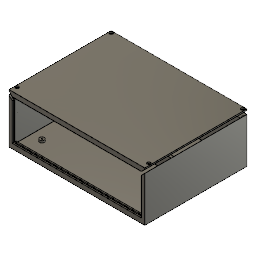
case_v1.26 (Autodesk Fusion 360 design; units mm, degrees)
Autodesk Fusion 360 part; units mm, degrees
sketch "bottom" plane through (0, 0, 0) normal (0, 1, 0) x (1, 0, 0)
  line L0 (-98.8893, -25.3823) -> (99.1107, -25.3823)
  line L1 (99.1107, -25.3823) -> (99.1107, -27.1323)
  line L2 (99.1107, -27.1323) -> (-98.8893, -27.1323)
  line L3 (-98.8893, -27.1323) -> (-98.8893, -25.3823)
  line L4 (-101.3893, 123.8677) -> (101.6107, 123.8677)
  line L5 (101.6107, 123.8677) -> (101.6107, -29.1323)
  line L6 (101.6107, -29.1323) -> (-101.3893, -29.1323)
  line L7 (-101.3893, -29.1323) -> (-101.3893, 123.8677)
  line L8 (-96.3893, 118.8677) -> (96.6107, 118.8677)
  line L9 (96.6107, 118.8677) -> (96.6107, -23.3823)
  line L10 (96.6107, -23.3823) -> (-96.3893, -23.3823)
  line L11 (-96.3893, -23.3823) -> (-96.3893, 118.8677)
  line L12 (96.6107, -23.3823) -> (96.6107, -25.3823)
  line L13 (96.6107, -27.1323) -> (96.6107, -29.1323)
  line L14 (-96.3893, -23.3823) -> (-96.3893, -25.3823)
  line L15 (-96.3893, -27.1323) -> (-96.3893, -29.1323)
  circle A0 centre (-79.3893, -1.6323) radius 3.5
  line L16 (-89.3893, 118.8677) -> (89.6107, 118.8677)
  line L17 (89.6107, 118.8677) -> (89.6107, 56.8677)
  line L18 (89.6107, 56.8677) -> (-89.3893, 56.8677)
  line L19 (-89.3893, 56.8677) -> (-89.3893, 118.8677)
  line L20 (0.1107, 123.8677) -> (0.1107, -29.1323) construction
  line L21 (93.6107, 118.8677) -> (93.6107, 52.8677)
  line L22 (93.6107, 52.8677) -> (-93.3893, 52.8677)
  line L23 (-93.3893, 52.8677) -> (-93.3893, 118.8677)
  circle A1 centre (0.1111, 37.8677) radius 3.5
  line L24 (96.6107, -23.3823) -> (101.6107, -23.3823) construction
  line L25 (96.6107, -23.3823) -> (101.6107, -23.3823) construction
  line L26 (96.6107, -23.3823) -> (103.6838, -23.3823) construction
  circle A2 centre (79.6107, -1.6323) radius 3.5
  dimension "d1" = 1.75
  dimension "d2" = 198
  dimension "d3" = 2.5
  dimension "d4" = 2.5
  dimension "d5" = 2
  dimension "d6" = 5
  dimension "d7" = 2
  dimension "d8" = 5
  dimension "d9" = 5
  dimension "d14" = 5
  dimension "d15" = 5
  dimension "d26" = 7
  dimension "d31" = 62
  dimension "d33" = 179
  dimension "d34" = 4
  dimension "d35" = 80
  dimension "d40" = 25.5
  dimension "d41" = 17
  dimension "d43" = 7
  dimension "d44" = 65
  dimension "d65" = 7
  measures "d1" distance of L0 L2
  measures "d2" distance of L1 L3
  measures "d3" distance of L3 L7
  measures "d4" distance of L1 L5
  measures "d5" distance of L2 L6
  measures "d6" distance of L5 L9
  measures "d7" distance of L0 L10
  measures "d8" distance of L7 L11
  measures "d9" distance of L4 L8
  measures "d14" distance of L5 L13
  measures "d15" distance of L7 L15
  measures "d26" diameter of A0
  measures "d31" distance of L16 L18
  measures "d33" distance of L17 L19
  measures "d35" distance of L2 L22
  measures "d43" diameter of A1
  measures "d65" diameter of A2
extrude "groundplane_extrude" add sketch "bottom" along normal blind 5 contours L8 L9 L10 L11 L21 L22 L23 | L8 L17 L18 L19 L21 L22 L23 | L8 L16 L17 L18 L19 | A0 | A1 | A2 makes body 1
extrude "front_lip_extrude" add sketch "bottom" along normal blind 7.5 contours L0 L10 L12 L14 | L2 L6 L13 L15 bodies 1 makes body 2 at (32.2774, 2.5, 27.1323)
extrude "front_lip_inner_extrude" add sketch "bottom" along normal blind 5 contours L0 L1 L2 L3 bodies 1 2
extrude "side_wall_extrude" add sketch "bottom" along normal blind 67.5 contours L0 L1 L2 L3 L4 L5 L6 L7 L8 L9 L11 L12 L13 L14 L15 L16 bodies 1
extrude "battery_compartment_extrude" add sketch "bottom" along normal blind 25 contours L8 L17 L18 L19 L21 L22 L23 bodies 1
extrude "extrude_pcb_mounts" add sketch "bottom" along normal blind 8 contours A0 | A1 | A2 bodies 1
hole "left_pcb_hole" at (-79.3893, 8, 1.6323) direction (0, -1, 0) diameter 2.3 depth 5 tip angle 180 bodies 1
hole "center_pcb_hole" at (0.1111, 8, -37.8677) direction (0, -1, 0) diameter 2.3 depth 5 tip angle 180 bodies 1
hole "right_pcb_hole" at (79.6107, 8, 1.6323) direction (0, -1, 0) diameter 2.3 depth 5 tip angle 180 bodies 1
sketch "top" plane through (0, 67.5, 0) normal (0, 1, 0) x (-1, 0, 0)
  line L0 (98.8893, 27.1323) -> (98.8893, 25.3823)
  line L1 (98.8893, 25.3823) -> (96.3893, 25.3823)
  line L2 (96.3893, 25.3823) -> (96.3893, -118.8677)
  line L3 (96.3893, -118.8677) -> (-96.6107, -118.8677)
  line L4 (-96.6107, -118.8677) -> (-96.6107, 25.3823)
  line L5 (-96.6107, 25.3823) -> (-99.1107, 25.3823)
  line L6 (-99.1107, 25.3823) -> (-99.1107, 27.1323)
  line L7 (-99.1107, 27.1323) -> (-96.6107, 27.1323)
  line L8 (-96.6107, 27.1323) -> (-96.6107, 29.1323)
  line L9 (-96.6107, 29.1323) -> (-101.6107, 29.1323)
  line L10 (-101.6107, 29.1323) -> (-101.6107, -123.8677)
  line L11 (-101.6107, -123.8677) -> (101.3893, -123.8677)
  line L12 (101.3893, -123.8677) -> (101.3893, 29.1323)
  line L13 (101.3893, 29.1323) -> (96.3893, 29.1323)
  line L14 (96.3893, 29.1323) -> (96.3893, 27.1323)
  line L15 (96.3893, 27.1323) -> (98.8893, 27.1323)
  line L16 (96.3893, -118.8677) -> (101.3893, -123.8677)
  line L17 (-0.1107, -123.8677) -> (-0.1107, 29.1323) construction
  line L18 (96.3893, -118.8677) -> (98.0863, -120.5648)
  line L19 (96.3893, 19.9724) -> (101.3905, 19.9724)
  line L20 (96.3893, 19.9724) -> (98.3893, 19.9724)
  line L21 (25, -75) -> (-25, -75)
  line L22 (-25, -75) -> (-25, -100)
  line L23 (-25, -100) -> (25, -100)
  line L24 (25, -100) -> (25, -75)
  dimension "d105" = 2.4
  dimension "d106" = 2
hole "Hole5" at (-98.3893, 67.5, 19.9724) direction (0, -1, 0) diameter 2.4 depth 25 tip angle 180 bodies 1
hole "Hole6" at (-98.0863, 67.5, -120.5648) direction (0, -1, 0) diameter 2.4 depth 25 tip angle 180 bodies 1
hole "Hole7" at (98.3078, 67.5, -120.5648) direction (0, -1, 0) diameter 2.4 depth 25 tip angle 180 bodies 1
hole "Hole8" at (98.6107, 67.5, 19.9724) direction (0, -1, 0) diameter 2.4 depth 25 tip angle 180 bodies 1
extrude "cover_brim" add 1 faces at (-32.3865, 67.5, -123.0903) along direction (0, 1, 0) blind 7 separate body on bodies 1 makes body 3
extrude "Extrude18" add 2 faces at (-96.3893, 69.8333, 27.7989) (-96.3893, 69.8333, -22.7011) along direction (1, 0, 0) blind 193 on bodies 3 bodies 3
sketch "Sketch3" plane through (0, 0, 29.1323) normal (0, 0, 1) x (1, 0, 0)
  line L0 (-101.3893, 67.5) -> (101.6107, 67.5)
  line L1 (101.6107, 67.5) -> (101.6107, 74.5)
  line L2 (101.6107, 74.5) -> (-101.3893, 74.5)
  line L3 (-101.3893, 74.5) -> (-101.3893, 67.5)
  line L4 (-101.3893, 71) -> (101.6107, 71)
extrude "Extrude19" add sketch "Sketch3" against normal blind 5 contours L1 L2 L3 L4 bodies 3
chamfer "Chamfer3" distance 5 angle 45 4 edges at (-96.3893, 67.5, -46.7427) (-96.3893, 67.5, 28.1323) (0.1107, 67.5, -118.8677) (96.6107, 67.5, -46.7427) on bodies 1
chamfer "Chamfer4" distance 5 angle 45 3 edges at (-101.3893, 67.5, -47.3677) (0.1107, 67.5, -123.8677) (101.6107, 67.5, -47.3677) on bodies 3
hole "Hole9" at (-98.3893, 74.5, 19.9724) direction (0, -1, 0) diameter 5 depth 2 tip angle 180 bodies 3
hole "Hole10" at (-98.0863, 74.5, -120.5648) direction (0, -1, 0) diameter 5 depth 2 tip angle 180 bodies 3
hole "Hole11" at (98.3078, 74.5, -120.5648) direction (0, -1, 0) diameter 5 depth 2 tip angle 180 bodies 3
hole "Hole12" at (98.6107, 74.5, 19.9724) direction (0, -1, 0) diameter 5 depth 2 tip angle 180 bodies 3
extrude "Extrude20" add sketch "top" against normal blind 19.5 contours L21 L22 L23 L24 bodies 3
named bodies: "case", "lid"
